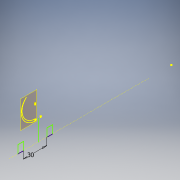
# Autodesk Inventor part: 長方形塊
Saved by Autodesk Inventor 2017 (Build 210142000, 142)
## iProperties
Part Number: 長方形塊
Material: 一般
Document SubType Name: Modeling
Designer: 士正
Density: 1 g/cm^3
Appearance: 預設
Author: 士正
Autodesk Inventor part; units mm, degrees
ref_plane "YZ Plane" through (0, 0, 0) normal (1, 0, 0) x (0, 1, 0)
ref_plane "XZ Plane" through (0, 0, 0) normal (0, 1, 0) x (-1, 0, 0)
ref_plane "工作平面1" through (125.3258, -174.2563, 26.6747) normal (1, 0, 0) x (0, 1, 0)
sketch "草圖1" plane through (125.3258, -174.2563, 26.6747) normal (1, 0, 0) x (0, 1, 0)
  arc A0 (0, -1.1604) -> (0, 1.1604) centre (0, 0) ccw projected
  arc A1 (-11.4249, 30.749) -> (0, 1.1604) centre (0, 18.1604) ccw projected
  arc A2 (-11.4249, 30.749) -> (0, -1.1604) centre (0, 16.8396) ccw projected
  line L0 (146.0063, -26.6747) -> (-33.9937, -26.6747) construction
  line L1 (-21.5, -26.6747) -> (-11.5, -26.6747)
  line L2 (-11.5, -26.6747) -> (-11.5, -11.6747)
  line L3 (-11.5, -11.6747) -> (-21.5, -11.6747)
  line L4 (-21.5, -11.6747) -> (-21.5, -26.6747)
  line L5 (18.5, -26.6747) -> (28.5, -26.6747)
  line L6 (28.5, -26.6747) -> (28.5, -11.6747)
  line L7 (28.5, -11.6747) -> (18.5, -11.6747)
  line L8 (18.5, -11.6747) -> (18.5, -26.6747)
  circle A3 centre (7, 0.0707) radius 1.1024 projected
  line L9 (3.5, 0) -> (3.5, -26.6747) construction
  point P0 (174.2563, -26.6747)
  dimension "d0" = 30
  dimension "d1" = 3.5
  dimension "d2" = 10
  dimension "d3" = 15
  constraints: 18 end point, 4 parallel, 3 perpendicular, 3 point on line, 2 collinear, 2 horizontal, 1 horizontal alignment, 1 other
  measures "d0" distance between parallel lines of L2 L8
  measures "d1" horizontal distance of L9.start A3.centre
  measures "d2" distance of L6.end L7.end
  measures "d3" distance of L3.end L1.start
ref_plane "工作平面2" through (-183.1603, -208.25, 0) normal (1, 0, 0) x (0, 1, 0)
extrude "擠出1" add sketch "草圖1" against normal up to surface (308.4861 mm away) contours L4 L3 L2 L1 | L8 L7 L6 L5
